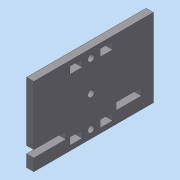
# Autodesk Inventor part: X-Anchor_Front-Side
Saved by Autodesk Inventor 2016 SP1 (Build 200210100, 210)
## iProperties
Created: 2016-03-02
Part Number: X-Anchor_Front-Side
Material: Generic
Document SubType Name: Modeling
Designer: Mohamed A.
Density: 1 g/cm^3
Appearance: Default
Author: Mohamed A.
Autodesk Inventor part; units mm, degrees
ref_plane "YZ Plane" through (0, 0, 0) normal (1, 0, 0) x (0, 1, 0)
ref_plane "XZ Plane" through (0, 0, 0) normal (0, 1, 0) x (-1, 0, 0)
ref_plane "XY Plane" through (0, 0, 0) normal (0, 0, 1) x (1, 0, 0)
sketch "Sketch2" plane through (0, 0, 0) normal (1, 0, 0) x (0, 1, 0)
  line L0 (-22.5, -21.5) -> (27.5, -21.5)
  line L1 (27.5, -21.5) -> (27.5, 11.2265)
  line L2 (27.5, 11.2265) -> (-22.5, 11.2265)
  line L3 (-22.5, 11.2265) -> (-22.5, 0)
  line L4 (-22.5, -21.5) -> (-22.5, -16.5)
  line L5 (-32.5, 0) -> (37.5, 0) construction
  line L6 (10.5, -19.5) -> (5.25, -19.5) projected
  line L7 (5.25, -19.5) -> (5.25, -16.5) projected
  line L8 (10.5, -16.5) -> (5.25, -16.5) projected
  line L9 (10.5, -19.5) -> (10.5, -16.5) projected
  line L10 (-2.25, -19.5) -> (-7.5, -19.5) projected
  line L11 (-7.5, -19.5) -> (-7.5, -16.5) projected
  line L12 (-2.25, -16.5) -> (-7.5, -16.5) projected
  line L13 (-2.25, -19.5) -> (-2.25, -16.5) projected
  line L14 (-9, -13.5) -> (-22.5, -13.5) projected
  line L15 (-9, -13.5) -> (-9, -16.5) projected
  line L16 (-22.5, -16.5) -> (-9, -16.5) projected
  line L17 (-22.5, -13.5) -> (-22.5, -16.5) projected
  line L18 (22.5, -13.5) -> (12, -13.5) projected
  line L19 (22.5, -13.5) -> (22.5, -16.5) projected
  line L20 (12, -16.5) -> (22.5, -16.5) projected
  line L21 (12, -13.5) -> (12, -16.5) projected
  line L22 (10.5, 6.2265) -> (5.25, 6.2265) projected
  line L23 (5.25, 6.2265) -> (5.25, 9.2265) projected
  line L24 (10.5, 9.2265) -> (5.25, 9.2265) projected
  line L25 (10.5, 6.2265) -> (10.5, 9.2265) projected
  line L26 (-2.25, 6.2265) -> (-7.5, 6.2265) projected
  line L27 (-7.5, 6.2265) -> (-7.5, 9.2265) projected
  line L28 (-2.25, 9.2265) -> (-7.5, 9.2265) projected
  line L29 (-2.25, 6.2265) -> (-2.25, 9.2265) projected
  line L30 (-22.5, -13.5) -> (-22.5, 0)
  line L31 (-22.5, -16.5) -> (-22.5, -13.5)
  line L32 (5.25, 9.2265) -> (-2.25, 6.2265) construction
  line L33 (-2.25, 9.2265) -> (5.25, 6.2265) construction
  line L34 (5.25, -16.5) -> (-2.25, -19.5) construction
  line L35 (-2.25, -16.5) -> (5.25, -19.5) construction
  circle A0 centre (1.5, 7.7265) radius 1.4
  circle A1 centre (1.5, -18) radius 1.4
  line L36 (1.5, 7.7265) -> (1.5, -18) construction
  circle A2 centre (1.5, -5.1367) radius 1.4
  dimension "d21" = 2
  dimension "d22" = 2
  dimension "d23" = 5
  dimension "d24" = 2.8
  dimension "d25" = 2.8
  dimension "d26" = 2.8
  constraints: 26 end point, 3 centre point, 3 midpoint, 3 perpendicular, 2 parallel, 1 collinear, 1 point on line, 1 vertical
  measures "d21" distance between parallel lines of L10 L0
  measures "d22" distance between parallel lines of L28 L2
  measures "d23" distance between parallel lines of L19 L1
  measures "d24" diameter of A0
  measures "d25" diameter of A1
  measures "d26" diameter of A2
extrude "Extrusion1" add sketch "Sketch2" along normal blind 3 contours L4 L16 L15 L14 L30 L3 L2 L1 L0
body "Solid1"
